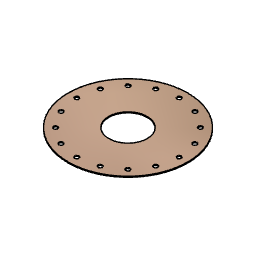
shield connector v5 (Autodesk Fusion 360 design; units mm, degrees)
Autodesk Fusion 360 part; units mm, degrees
note: some values were not read from the file. Set by a fixed rule: the direction of a hole.
sketch "Sketch1" plane through (0, 0, 0) normal (0, 1, 0) x (1, 0, 0)
  circle A0 centre (0, 0) radius 60 construction
  circle A1 centre (0, 0) radius 22.5
  circle A2 centre (0, 0) radius 70
  point P0 (-60, 0)
  dimension "d1" = 120
  dimension "d2" = 45
  dimension "d3" = 140
  constraint coincident A0.centre A1.centre
  constraint concentric A0 A1
  constraint coincident A0 P0
  constraint horizontal A0.centre P0
  measures "d1" diameter of A0
  measures "d2" diameter of A1
  measures "d3" diameter of A2
extrude "Extrude1" add sketch "Sketch1" along normal blind 1
hole "Hole1" at (-60, 0, 0) direction (0, 1, 0) diameter 5 depth 30 tip angle 118
pattern_circular "C-Pattern1" count 16 over 360 about axis through (0, 1.75, 0) along (0, 1, 0) of "Hole1"
sketch "cutting pattern" plane through (0, 1, 0) normal (0, 1, 0) x (-1, 0, 0)
  circle A0 centre (55.4328, -22.961) radius 2.5
  circle A1 centre (42.4264, -42.4264) radius 2.5
  circle A2 centre (22.961, -55.4328) radius 2.5
  circle A3 centre (0, -60) radius 2.5
  circle A4 centre (-22.961, -55.4328) radius 2.5
  circle A5 centre (-42.4264, -42.4264) radius 2.5
  circle A6 centre (-55.4328, -22.961) radius 2.5
  circle A7 centre (-60, 0) radius 2.5
  circle A8 centre (-55.4328, 22.961) radius 2.5
  circle A9 centre (-42.4264, 42.4264) radius 2.5
  circle A10 centre (-22.961, 55.4328) radius 2.5
  circle A11 centre (0, 60) radius 2.5
  circle A12 centre (22.961, 55.4328) radius 2.5
  circle A13 centre (42.4264, 42.4264) radius 2.5
  circle A14 centre (55.4328, 22.961) radius 2.5
  circle A15 centre (60, 0) radius 2.5
  circle A16 centre (0, 0) radius 22.5
  circle A17 centre (0, 0) radius 70
